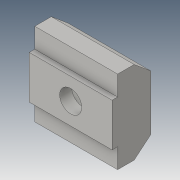
# Autodesk Inventor part: #6_8mm_tnut_adapter
Saved by Autodesk Inventor 2016 (Build 200138000, 138)
## iProperties
Created: 2017-05-10
Part Number: #6_8mm_tnut_adapter
Material: Generic
Document SubType Name: Modeling
Designer: Spark Electronics
Density: 1 g/cm^3
Appearance: Default
Author: Spark Electronics
Autodesk Inventor part; units mm, degrees
ref_plane "YZ Plane" through (0, 0, 0) normal (1, 0, 0) x (0, 1, 0)
ref_plane "XZ Plane" through (0, 0, 0) normal (0, 1, 0) x (-1, 0, 0)
ref_plane "XY Plane" through (0, 0, 0) normal (0, 0, 1) x (1, 0, 0)
sketch "Sketch1" plane through (0, 0, 0) normal (1, 0, 0) x (0, 1, 0)
  line L0 (4.9995, -3.5501) -> (-5.0005, -3.5501)
  line L1 (-7.5, -0.5501) -> (-7.5, 2.4499)
  line L2 (7.5, 2.4499) -> (7.5, -0.5501)
  line L3 (7.8075, -4.2648) -> (-4.4849, 2.4499) construction
  line L4 (-7.8075, -4.2648) -> (4.4849, 2.4499) construction
  line L5 (-5.0005, -3.5501) -> (-7.5, -0.5501)
  line L6 (4.9995, -3.5501) -> (7.5, -0.5501)
  line L7 (7.5, 2.4499) -> (-7.5, 2.4499)
  line L8 (-3.9, 3.4499) -> (3.9, 3.4499)
  line L9 (-2.6673, 1.4363) -> (-2.6673, 1.457)
  line L10 (-3.9, 2.4499) -> (-3.9, 3.4499)
  line L11 (3.9, 3.4499) -> (3.9, 2.4499)
  line L12 (2.6673, 1.457) -> (2.6673, 1.4363)
  line L13 (2.6673, 1.4363) -> (2.6295, 1.4363)
  line L14 (-2.6295, 1.4363) -> (-2.6673, 1.4363)
  line L15 (2.6673, 1.4363) -> (2.6446, 1.4446) construction
  line L16 (-2.6673, 1.4363) -> (-2.6446, 1.4446) construction
  line L17 (0, 0) -> (0, 11.1937)
  point P0 (0, 3.4499)
  point P1 (0, 2.4499)
  dimension "d0" = 15
  dimension "d1" = 3
  dimension "d2" = 3
  dimension "d5" = 10
  dimension "d6" = 129.8
  dimension "d7" = 7.8
  dimension "d8" = 1
  dimension "d9" = 6
  constraints: 36 end point, 13 point on line, 7 parallel, 6 perpendicular, 3 horizontal, 2 midpoint, 1 vertical
  measures "d0" distance between parallel lines of L2 L1
  measures "d1" distance of L2.start L2.end
  measures "d2" distance of L1.start L1.end
  measures "d5" distance of L0.start L0.end
  measures "d6" angle of L5 L0
  measures "d7" distance of L8.start L8.end
  measures "d8" distance of L10.start L8.start
  measures "d9" distance between parallel lines of L0 L7
extrude "Extrusion1" add sketch "Sketch1" along normal blind 15
sketch "Sketch2" plane through (0, -5.0005, -3.5501) normal (0, 0, -1) x (-1, 0, 0)
  line L0 (-3.4, 3.3022) -> (-5.8017, 0.9005)
  line L1 (-5.8017, 0.9005) -> (-9.1983, 0.9005)
  line L2 (-9.1983, 0.9005) -> (-11.6, 3.3022)
  line L3 (-11.6, 3.3022) -> (-11.6, 6.6988)
  line L4 (-11.6, 6.6988) -> (-9.1983, 9.1005)
  line L5 (-9.1983, 9.1005) -> (-5.8017, 9.1005)
  line L6 (-5.8017, 9.1005) -> (-3.4, 6.6988)
  line L7 (-3.4, 6.6988) -> (-3.4, 3.3022)
  line L8 (0, 0) -> (0, 10) projected
  line L9 (0, 12.5005) -> (-15, 12.5005) projected
  point P0 (0, 3.9)
  point P1 (-7.5, 5.0005)
  point P2 (15, 12.4675)
  point P3 (15, 12.4675)
  dimension "d12" = 8.2
  dimension "d25" = 7.5
  dimension "d26" = 7.5
  constraints: 16 end point, 1 coincident, 19 other
  measures "d12" distance between parallel lines of L3 L7
  measures "d25" distance from line of point (-7.5, 5) L8
  measures "d26" distance from line of L9 point (-7.5, 5)
extrude "Extrusion2" cut sketch "Sketch2" against normal blind 4.8
hole "Hole2" at (7.5, 0, 1.2499) direction (0, 0, 1) diameter 4 end through all
body "Solid1"
